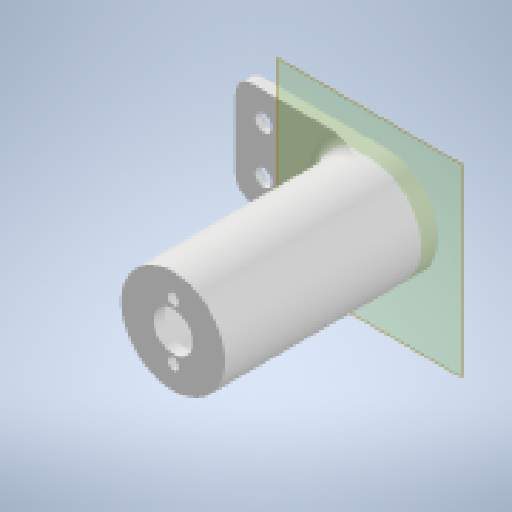
# Autodesk Inventor part: Camisa Motor
Saved by Autodesk Inventor 2023 (Build 270158000, 158)
## iProperties
Created: 2023-04-20
Part Number: Camisa Motor
Material: Genérico
Document SubType Name: Modeling
Designer: sergi
Density: 1 g/cm^3
Appearance: Valor por defecto
Author: sergi
Autodesk Inventor part; units mm, degrees
ref_plane "YZ Plane" through (0, 0, 0) normal (1, 0, 0) x (0, 1, 0)
ref_plane "XZ Plane" through (0, 0, 0) normal (0, 1, 0) x (-1, 0, 0)
ref_plane "Plano de trabajo1" through (-97, 17, -59.7) normal (0, 0, -1) x (0, 1, 0)
sketch "Boceto1" plane through (0, 0, 0) normal (0, 0, 1) x (1, 0, 0)
  circle A0 centre (0, -5) radius 1 projected
  circle A1 centre (0, 5) radius 1 projected
  circle A2 centre (0, 0) radius 3.5 projected
  circle A3 centre (0, 0) radius 8 projected
  circle A4 centre (0, 0) radius 8.5
  circle A5 centre (0, 0) radius 9.25
  dimension "d0" = 17
  dimension "d1" = 18.5
  constraints: 2 centre point, 2 coincident
  measures "d0" diameter of A4
  measures "d1" diameter of A5
extrude "Extrusión1" add sketch "Boceto1" against normal blind 36.2 contours A5
sketch "Boceto2" plane through (0, 0, 0) normal (0, 0, 1) x (1, 0, 0)
  circle A0 centre (0, 0) radius 9.25
  circle A1 centre (0, -5) radius 1 projected
  circle A2 centre (0, 5) radius 1 projected
  circle A3 centre (0, 0) radius 3.5 projected
  circle A4 centre (0, 0) radius 8 projected
  constraints: 1 centre point, 1 coincident
extrude "Extrusión2" add sketch "Boceto2" along normal blind 2 contours A0 | A4
ref_plane "Plano de trabajo2" through (0, 0, -33.2) normal (0, 0, -1) x (-1, 0, 0)
sketch "Boceto10" plane through (0, 0, -36.2) normal (0, 0, -1) x (-1, 0, 0)
  circle A0 centre (0, 0) radius 9.25 projected
  line L0 (0, 9.25) -> (25, 9.25)
  line L1 (25, 9.25) -> (25, -9.25)
  line L2 (25, -9.25) -> (0, -9.25)
  line L3 (0, -9.25) -> (0, 9.25)
  dimension "d43" = 25
  dimension "d44" = 18.5
  constraints: 8 end point, 2 parallel, 1 horizontal, 1 perpendicular, 2 other
  measures "d43" distance of L1.end L2.end
  measures "d44" distance of L0.end L1.end
extrude "Extrusión7" add sketch "Boceto10" against normal blind 2 contours A0 L0 L1 L2
fillet "Empalme4" radius 3 1 edges at (-9.25, 0, -34.2)
sketch "Boceto11" plane through (0, 0, -36.2) normal (0, 0, -1) x (-1, 0, 0)
  line L0 (25, -9.25) -> (25, 9.25) projected
  line L1 (25, 9.25) -> (0, 9.25) projected
  line L2 (0, -9.25) -> (25, -9.25) projected
  point P0 (0, 0)
  point P1 (20, 4.25)
  point P2 (20, -4.25)
  dimension "d48" = 5
  dimension "d49" = 5
  dimension "d50" = 5
  dimension "d51" = 5
  measures "d48" distance from line of L0 point (20, 4.25)
  measures "d49" distance from line of L1 point (20, 4.25)
  measures "d50" distance from line of L0 point (20, -4.25)
  measures "d51" distance from line of L2 point (20, -4.25)
hole "Agujero2" at (-20, 4.25, -36.2) at (-20, -4.25, -36.2) direction (0, 0, 1) diameter 3 end through all countersink diameter 5 countersink angle 90
fillet "Empalme5" radius 3 2 edges at (-25, 9.25, -35.2) (-25, -9.25, -35.2)
